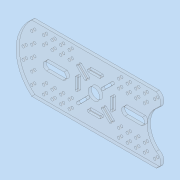
# Autodesk Inventor part: 底盘设计1.2
Saved by Autodesk Inventor 2019 (Build 230136000, 136)
## iProperties
Created: 2020-10-19
Part Number: 底盘设计1.2
Material: 聚碳酸酯，透明
Document SubType Name: Modeling
Designer: Wang Hua
Density: 1.2 g/cm^3
Appearance: 聚碳酸酯 - 透明
Author: Wang Hua
Autodesk Inventor part; units mm, degrees
ref_plane "YZ Plane" through (0, 0, 0) normal (1, 0, 0) x (0, 1, 0)
ref_plane "XZ Plane" through (0, 0, 0) normal (0, 1, 0) x (-1, 0, 0)
ref_plane "XY Plane" through (0, 0, 0) normal (0, 0, 1) x (1, 0, 0)
sketch "草图1" plane through (0, 0, 0) normal (0, 0, 1) x (1, 0, 0)
  line L0 (80, -42.5) -> (-80, -42.5)
  line L1 (-80, 42.5) -> (80, 42.5)
  line L2 (80, -42.5) -> (-80, 42.5) construction
  line L3 (-80, -42.5) -> (80, 42.5) construction
  arc A0 (-80, 42.5) -> (-80, -42.5) centre (-45.0894, 0) ccw
  line L4 (0, 50.4113) -> (0, -46.1071) construction
  line L5 (96.3853, 0) -> (-113.3157, 0) construction
  line L6 (0, 24) -> (80, 24) construction
  line L7 (-155.9274, 0) -> (142.3547, 0) construction
  arc A1 (80, 24) -> (80, -24) centre (99.7429, 0) ccw
  arc A2 (80, 24) -> (80, 42.5) centre (75.8823, 33.25) ccw
  arc A3 (80, -42.5) -> (80, -24) centre (75.8823, -33.25) ccw
  circle A4 centre (0, 0) radius 7.5
  line L8 (0, 0) -> (-30.1738, 30.1738) construction
  arc A5 (-21.2132, 21.2132) -> (-20.0949, 22.2754) centre (0, 0) ccw construction
  arc A6 (-11.6306, 9.4725) -> (-9.4725, 11.6306) centre (0, 0) ccw construction
  line L9 (-10.6066, 10.6066) -> (-11.7026, 9.5106) construction
  circle A7 centre (0, 0) radius 22.5 construction
  line L10 (-20.1172, 22.3092) -> (-9.5106, 11.7026)
  line L11 (-10.6066, 10.6066) -> (-11.7026, 9.5106) construction
  line L12 (-11.7026, 9.5106) -> (-22.3092, 20.1172)
  line L13 (-20.1172, 22.3092) -> (-11.7026, 9.5106) construction
  line L14 (-9.5106, 11.7026) -> (-22.3092, 20.1172) construction
  arc A8 (-20.1172, 22.3092) -> (-22.3092, 20.1172) centre (-20.9053, 20.9053) ccw
  line L15 (-15.9099, 15.9099) -> (-9.5106, 22.3092) construction
  arc A9 (-11.7026, 9.5106) -> (-9.5106, 11.7026) centre (-10.9145, 10.9145) ccw
  line L16 (-24.05, -7.5) -> (-24.05, 7.5)
  line L17 (-20.95, 7.5) -> (-20.95, -7.5)
  line L18 (-20.95, -7.5) -> (-24.05, 7.5) construction
  line L19 (-24.05, -7.5) -> (-20.95, 7.5) construction
  arc A10 (-20.95, 7.5) -> (-24.05, 7.5) centre (-22.5, 7.0646) ccw
  arc A11 (-24.05, -7.5) -> (-20.95, -7.5) centre (-22.5, -7.0646) ccw
  line L20 (-31.8198, 0) -> (-31.8198, 22) construction
  line L21 (-31.8198, 22) -> (-64.8198, 22) construction
  line L22 (-31.8198, 22) -> (-31.8198, 33) construction
  line L23 (-31.8198, 33) -> (-64.8198, 33) construction
  line L24 (-39.9788, -4.6927) -> (-61.0474, -4.6927)
  line L25 (-62.4271, 5.3073) -> (-38.5991, 5.3073)
  line L26 (-39.9788, -4.6927) -> (-62.4271, 5.3073) construction
  line L27 (-61.0474, -4.6927) -> (-38.5991, 5.3073) construction
  arc A12 (-62.4271, 5.3073) -> (-61.0474, -4.6927) centre (-60.2132, 0.5176) ccw
  line L28 (-50.5131, 0) -> (-50.5131, 11.6306) construction
  arc A13 (-39.9788, -4.6927) -> (-38.5991, 5.3073) centre (-40.813, 0.5176) ccw
  line L29 (22.3092, 20.1172) -> (11.7026, 9.5106)
  line L30 (9.5106, 11.7026) -> (20.1172, 22.3092)
  arc A14 (22.3092, 20.1172) -> (20.1172, 22.3092) centre (20.9053, 20.9053) ccw
  arc A15 (9.5106, 11.7026) -> (11.7026, 9.5106) centre (10.9145, 10.9145) ccw
  line L31 (7.5, 20.95) -> (-7.5, 20.95)
  line L32 (-7.5, 24.05) -> (7.5, 24.05)
  arc A16 (7.5, 20.95) -> (7.5, 24.05) centre (7.0646, 22.5) ccw
  arc A17 (-7.5, 24.05) -> (-7.5, 20.95) centre (-7.0646, 22.5) ccw
  line L33 (20.1172, -22.3092) -> (9.5106, -11.7026)
  line L34 (11.7026, -9.5106) -> (22.3092, -20.1172)
  arc A18 (20.1172, -22.3092) -> (22.3092, -20.1172) centre (20.9053, -20.9053) ccw
  arc A19 (11.7026, -9.5106) -> (9.5106, -11.7026) centre (10.9145, -10.9145) ccw
  line L35 (20.95, -7.5) -> (20.95, 7.5)
  line L36 (24.05, 7.5) -> (24.05, -7.5)
  arc A20 (20.95, -7.5) -> (24.05, -7.5) centre (22.5, -7.0646) ccw
  arc A21 (24.05, 7.5) -> (20.95, 7.5) centre (22.5, 7.0646) ccw
  line L37 (-22.3092, -20.1172) -> (-11.7026, -9.5106)
  line L38 (-9.5106, -11.7026) -> (-20.1172, -22.3092)
  arc A22 (-22.3092, -20.1172) -> (-20.1172, -22.3092) centre (-20.9053, -20.9053) ccw
  arc A23 (-9.5106, -11.7026) -> (-11.7026, -9.5106) centre (-10.9145, -10.9145) ccw
  line L39 (-7.5, -20.95) -> (7.5, -20.95)
  line L40 (7.5, -24.05) -> (-7.5, -24.05)
  arc A24 (-7.5, -20.95) -> (-7.5, -24.05) centre (-7.0646, -22.5) ccw
  arc A25 (7.5, -24.05) -> (7.5, -20.95) centre (7.0646, -22.5) ccw
  line L41 (39.9788, -4.6927) -> (61.0474, -4.6927)
  line L42 (62.4271, 5.3073) -> (38.5991, 5.3073)
  arc A26 (61.0474, -4.6927) -> (62.4271, 5.3073) centre (60.2132, 0.5176) ccw
  arc A27 (38.5991, 5.3073) -> (39.9788, -4.6927) centre (40.813, 0.5176) ccw
  point P0 (-22.5, 0)
  point P1 (78.044, 33.25)
  point P2 (78.044, -33.25)
  point P3 (-53.8198, 22)
  point P4 (-42.8198, 22)
  point P5 (-53.8198, 33)
  point P6 (-42.8198, 33)
  point P7 (-80, 0)
  point P8 (-80, 15)
  point P9 (-80, 30)
  point P10 (-31.8198, -22)
  point P11 (-64.8198, -22)
  point P12 (-53.8198, -22)
  point P13 (-42.8198, -22)
  point P14 (-31.8198, -33)
  point P15 (-64.8198, -33)
  point P16 (-53.8198, -33)
  point P17 (-42.8198, -33)
  point P18 (-80, -15)
  point P19 (-80, -30)
  point P20 (31.8198, 22)
  point P21 (64.8198, 22)
  point P22 (53.8198, 22)
  point P23 (42.8198, 22)
  point P24 (31.8198, 33)
  point P25 (64.8198, 33)
  point P26 (53.8198, 33)
  point P27 (42.8198, 33)
  point P28 (31.8198, -33)
  point P29 (31.8198, -22)
  point P30 (42.8198, -33)
  point P31 (42.8198, -22)
  point P32 (53.8198, -33)
  point P33 (53.8198, -22)
  point P34 (64.8198, -33)
  point P35 (64.8198, -22)
  point P36 (-91.0115, 7.5)
  point P37 (11.6306, 9.4725)
  point P38 (9.4725, 11.6306)
  point P39 (9.4725, -11.6306)
  point P40 (11.6306, -9.4725)
  point P41 (-11.6306, -9.4725)
  point P42 (-9.4725, -11.6306)
  point P43 (-91.0115, -7.5)
  dimension "d0" = 160
  dimension "d1" = 24
  dimension "d2" = 85
  dimension "d3" = 15
  dimension "d4" = 45
  dimension "d5" = 60
  dimension "d6" = 30
  dimension "d7" = 1.55
  dimension "d8" = 45
  dimension "d9" = 3.1
  dimension "d10" = 15
  dimension "d11" = 1.61
  dimension "d12" = 1.61
  dimension "d13" = 22
  dimension "d15" = 11
  dimension "d16" = 11
  dimension "d17" = 11
  dimension "d18" = 33
  dimension "d19" = 55
  dimension "d20" = 15
  dimension "d21" = 15
  dimension "d22" = 10
  dimension "d25" = 7.5
  dimension "d28" = 360
  constraints: 84 end point, 62 point on circle, 28 centre point, 26 symmetric about line, 13 coincident, 13 vertical alignment, 11 point on line, 6 midpoint, 6 parallel, 5 horizontal, 4 vertical, 2 perpendicular, 2 tangent, 1 equal radius, 104 other
  measures "d0" distance of L1.start L1.end
  measures "d1" distance of the line from the sketch origin of L6
  measures "d2" distance between parallel lines of L0 L1
  measures "d3" diameter of A4
  measures "d4" angle of L5 L8
  measures "d5" diameter of A5
  measures "d6" diameter of A6
  measures "d7" distance of L9.start L9.end
  measures "d8" diameter of A7
  measures "d9" distance between parallel lines of L17 L16
  measures "d10" distance of L16.start L16.end
  measures "d11" radius of A8
  measures "d12" radius of A10
  measures "d13" distance of L20.start L20.end
  measures "d15" distance of point (-53.82, 22) point (-64.82, 22)
  measures "d16" distance of L20.end point (-42.82, 22)
  measures "d17" distance of L22.start L22.end
  measures "d18" distance of L22.end L23.end
  measures "d19" radius of A0
  measures "d20" distance of point (-80, 15) point (-80, 0)
  measures "d21" distance of point (-80, 30) point (-80, 15)
  measures "d22" distance between parallel lines of L24 L25
extrude "拉伸1" add sketch "草图1" along normal blind 4 contours L0 A0 L1 A2 A1 A3 | L29 A15 L30 A14 | L31 A17 L32 A16 | L33 A19 L34 A18 | L35 A21 L36 A20 | L37 A23 L38 A22 | L39 A25 L40 A24 | A27 L42 A26 L41
extrude "拉伸2" cut sketch "草图1" along normal through all contours L29 A15 L30 A14 | L31 A17 L32 A16 | L33 A19 L34 A18 | L35 A21 L36 A20 | L37 A23 L38 A22 | L39 A25 L40 A24
extrude "拉伸3" cut sketch "草图1" along normal through all contours A27 L42 A26 L41
hole "孔1" at (78.044, 33.25, 0) at (78.044, -33.25, 0) at (-31.8198, 22, 0) at (-64.8198, 22, 0) at (-53.8198, 22, 0) at (-42.8198, 22, 0) at (-31.8198, 33, 0) at (-64.8198, 33, 0) at (-53.8198, 33, 0) at (-42.8198, 33, 0) at (-80, 0, 0) at (-80, 15, 0) at (-80, 30, 0) at (-31.8198, -33, 0) at (-31.8198, -22, 0) at (-42.8198, -33, 0) at (-42.8198, -22, 0) at (-53.8198, -33, 0) at (-53.8198, -22, 0) at (-64.8198, -33, 0) at (-64.8198, -22, 0) at (-80, -30, 0) at (-80, -15, 0) at (42.8198, 22, 0) at (42.8198, 33, 0) at (53.8198, 33, 0) at (53.8198, 22, 0) at (64.8198, 22, 0) at (64.8198, -22, 0) at (53.8198, -22, 0) at (42.8198, -22, 0) at (31.8198, -22, 0) at (31.8198, -33, 0) at (42.8198, -33, 0) at (53.8198, -33, 0) at (64.8198, -33, 0) at (-91.0115, 7.5, 0) at (-91.0115, -7.5, 0) at (31.8198, 33, 0) at (31.8198, 22, 0) at (64.8198, 33, 0) direction (0, 0, 1) diameter 3.3 end through all
